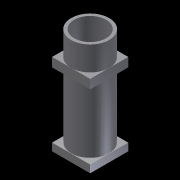
# Autodesk Inventor part: Sicherungshalter
Saved by Autodesk Inventor 2011 SP1 (Build 150282100, 282)
## iProperties
Created: 2012-07-12
Part Number: Sicherungshalter
Document SubType Name: Modeling
Designer: nfischer
Density: 1 g/cm^3
Author: nfischer
Autodesk Inventor part; units mm, degrees
ref_plane "YZ Plane" through (0, 0, 0) normal (1, 0, 0) x (0, 1, 0)
ref_plane "XZ Plane" through (0, 0, 0) normal (0, 1, 0) x (-1, 0, 0)
ref_plane "XY Plane" through (0, 0, 0) normal (0, 0, 1) x (1, 0, 0)
sketch "Skizze1" plane through (0, 0, 0) normal (0, 0, 1) x (1, 0, 0)
  line L0 (-6.3, 6.3) -> (6.3, 6.3)
  line L1 (6.3, 6.3) -> (6.3, -6.3)
  line L2 (6.3, -6.3) -> (-6.3, -6.3)
  line L3 (-6.3, -6.3) -> (-6.3, 6.3)
  circle A0 centre (0, 0) radius 6.3
  circle A1 centre (0, 0) radius 5.3
  circle A2 centre (0, 0) radius 5.3
  circle A3 centre (0, 0) radius 6.3
  point P0 (0, -6.3)
  point P1 (-6.3, 0)
  dimension "d0" = 12.6
  dimension "d1" = 12.6
  dimension "d23" = 10.6
  constraints: 8 end point, 6 coincident, 4 centre point, 2 concentric, 2 midpoint, 2 parallel, 1 horizontal, 1 horizontal alignment, 1 perpendicular, 1 tangent, 1 vertical alignment
  measures "d0" distance of L0.start L0.end
  measures "d1" distance of L2.end L0.start
  measures "d23" diameter of A1
extrude "Extrusion2" add sketch "Skizze1" along normal blind 3
sketch "Skizze2" plane through (0, 0, 3) normal (0, 0, 1) x (1, 0, 0)
  circle A0 centre (0, 0) radius 5.3 projected
  circle A1 centre (0, 0) radius 6.3
  dimension "d7" = 12.6
  constraints: 1 centre point, 1 coincident
  measures "d7" diameter of A1
extrude "Extrusion3" add sketch "Skizze2" along normal blind 8
sketch "Skizze3" plane through (0, 0, 0) normal (0, 0, -1) x (-1, 0, 0)
  circle A0 centre (0, 0) radius 5.3 projected
  circle A1 centre (0, 0) radius 5.3
  circle A2 centre (0, 0) radius 6.25
  dimension "d10" = 12.5
  constraints: 2 centre point, 2 coincident, 1 concentric
  measures "d10" diameter of A2
extrude "Extrusion4" add sketch "Skizze3" along normal blind 24
sketch "Skizze4" plane through (0, 0, -24) normal (0, 0, -1) x (-1, 0, 0)
  circle A0 centre (0, 0) radius 6.25 projected
  circle A1 centre (0, 0) radius 5.3 projected
  line L0 (-6.35, -6.35) -> (6.25, -6.35)
  line L1 (6.25, -6.35) -> (6.25, 6.25)
  line L2 (6.25, 6.25) -> (-6.35, 6.25)
  line L3 (-6.35, 6.25) -> (-6.35, -6.35)
  dimension "d25" = 10.6
  dimension "d26" = 12.5
  dimension "d29" = 12.6
  dimension "d30" = 12.6
  constraints: 8 end point, 2 parallel, 1 horizontal, 1 perpendicular
  measures "d25" diameter of A1
  measures "d26" diameter of A0
  measures "d29" distance of L1.end L2.end
  measures "d30" distance of L0.end L1.end
sketch "Skizze5" plane through (6.3, 6.3, 3) normal (0, 1, 0) x (1, 0, 0)
  point P0 (-6.75, 1.5)
hole "Hole1" at (-0.45, 6.3, 1.5) direction (0, -1, 0) diameter 2 depth 8 tip angle 118
extrude "Extrusion6" add sketch "Skizze4" against normal blind 2.5 contours L1 L0 L3 L2 A0 | A0 L2 L1
